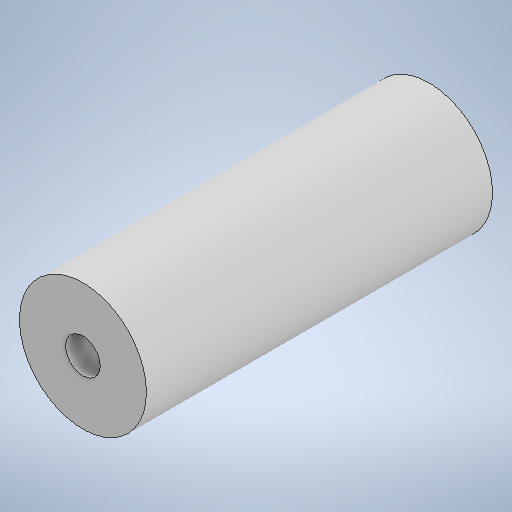
# Autodesk Inventor part: Shaft Coupler
Saved by Autodesk Inventor 2026.1 (Build 301233020, 233B)
## iProperties
Created: 2025-10-22
Part Number: Shaft Coupler
Material: Generic
Document SubType Name: Modeling
Designer: yo
Density: 1 g/cm^3
Appearance: Default
Author: yo
Autodesk Inventor part; units mm, degrees
ref_plane "YZ Plane" through (0, 0, 0) normal (1, 0, 0) x (0, 1, 0)
ref_plane "XZ Plane" through (0, 0, 0) normal (0, 1, 0) x (-1, 0, 0)
ref_plane "XY Plane" through (0, 0, 0) normal (0, 0, 1) x (1, 0, 0)
sketch "Sketch1" plane through (0, 0, 0) normal (0, 0, 1) x (1, 0, 0)
  circle A0 centre (0, 0) radius 1.5
  circle A1 centre (0, 0) radius 5.5
  circle A2 centre (0, 0) radius 3.5
  dimension "d0" = 3
  dimension "d1" = 11
  dimension "d2" = 7
  constraints: 3 centre point, 3 coincident
  measures "d0" diameter of A0
  measures "d1" diameter of A1
  measures "d2" diameter of A2
extrude "Extrusion1" add sketch "Sketch1" along normal mid plane 30 contours A1
extrude "Extrusion2" add sketch "Sketch1" along normal blind 15 contours A2
extrude "Extrusion3" add sketch "Sketch1" along normal mid plane 5 contours A0
extrude "Extrusion4" add sketch "Sketch1" against normal blind 2.5 contours A2
body "Solid1"
